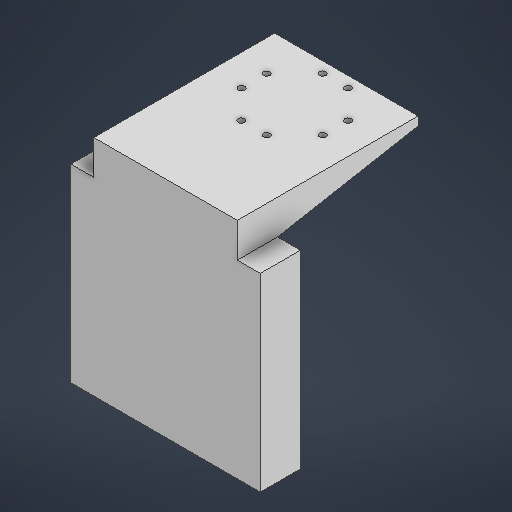
# Autodesk Inventor part: pan_base_holder_third
Saved by Autodesk Inventor 2026 (Build 300175000, 175)
## iProperties
Created: 2025-06-27
Part Number: pan_base_holder_third
Material: Generic
Document SubType Name: Modeling
Designer: user
Density: 1 g/cm^3
Appearance: Default
Author: user
Autodesk Inventor part; units mm, degrees
ref_plane "YZ Plane" through (0, 0, 0) normal (1, 0, 0) x (0, 1, 0)
ref_plane "XZ Plane" through (0, 0, 0) normal (0, 1, 0) x (-1, 0, 0)
ref_plane "XY Plane" through (0, 0, 0) normal (0, 0, 1) x (1, 0, 0)
sketch "Sketch1" plane through (0, 0, 0) normal (0, 0, 1) x (1, 0, 0)
  line L0 (-31, -31) -> (31, -31)
  line L1 (31, -31) -> (31, 31)
  line L2 (31, 31) -> (-31, 31)
  line L3 (-31, 31) -> (-31, -31)
  line L4 (-31, -31) -> (31, 31) construction
  line L5 (31, -31) -> (-31, 31) construction
  line L6 (-33, 33) -> (33, 33)
  line L7 (33, 33) -> (33, -33)
  line L8 (33, -33) -> (-33, -33)
  line L9 (-33, -33) -> (-33, 33)
  point P0 (0, 0)
  dimension "d0" = 62
  dimension "d1" = 62
  dimension "d2" = 2
  constraints: 20 end point, 4 parallel, 2 midpoint, 2 perpendicular, 1 horizontal, 3 other
  measures "d0" distance of L1.end L2.end
  measures "d1" distance of L0.end L1.end
  measures "d2" distance between parallel lines of L2 L6
extrude "Extrusion1" add sketch "Sketch1" along normal blind 2 contours L3 L2 L1 L0 | L6 L7 L8 L9
extrude "Extrusion2" add sketch "Sketch1" against normal blind 12
sketch "Sketch2" plane through (-33, 33, 2) normal (0, 1, 0) x (1, 0, 0)
  line L0 (8, 3) -> (58, 3)
  line L1 (58, 3) -> (58, 0)
  line L2 (58, 0) -> (8, 0)
  line L3 (8, 0) -> (8, 3)
  line L4 (0, 14) -> (0, 0) projected
  line L5 (0, 14) -> (66, 14) projected
  point P0 (33, 2)
  dimension "d7" = 50
  dimension "d8" = 3
  dimension "d9" = 8
  dimension "d10" = 11
  constraints: 8 end point, 2 parallel, 1 horizontal, 1 perpendicular
  measures "d7" distance of L1.end L2.end
  measures "d8" distance of L0.end L1.end
  measures "d9" distance between parallel lines of L4 L3
  measures "d10" distance between parallel lines of L5 L0
extrude "Extrusion3" add sketch "Sketch2" along normal blind 12
sketch "Sketch3" plane through (25, 33, -1) normal (0, 0, -1) x (-1, 0, 0)
  line L0 (50, 12) -> (0, 12) projected
  line L1 (50, 0) -> (50, 12) projected
  line L2 (0, 12) -> (50, 12)
  line L3 (50, 12) -> (50, 9)
  line L4 (50, 9) -> (0, 9)
  line L5 (0, 9) -> (0, 12)
  point P0 (25, -33)
  dimension "d13" = 3
  constraints: 8 end point, 2 parallel, 1 horizontal, 1 perpendicular, 1 point on line
  measures "d13" distance of L2.end L3.end
extrude "Extrusion4" add sketch "Sketch3" along normal blind 60
sketch "Sketch8" plane through (-25, 33, -1) normal (-1, 0, 0) x (0, 0, 1)
  line L0 (0, 9) -> (-60, 9) projected
  line L1 (0, 9) -> (-60, 9)
  line L2 (-60, 9) -> (-60, 0)
  line L3 (-60, 0) -> (0, 0)
  line L4 (0, 0) -> (0, 9)
  line L5 (-60, 9) -> (-10.9892, 0)
  point P0 (1, -33)
  dimension "d43" = 9
  constraints: 10 end point, 2 parallel, 1 horizontal, 1 perpendicular, 1 point on line
  measures "d43" distance of L2.end L1.end
extrude "Extrusion9" add sketch "Sketch8" against normal blind 2 contours L4 L3 L5 L0
ref_plane "Work Plane1" through (0, 33, 2) normal (1, 0, 0) x (0, 0, -1)
mirror "Mirror1" about plane through (0, 33, 2) normal (1, 0, 0) of "Extrusion9"
sketch "Sketch9" plane through (-33, 45, 2) normal (0, 1, 0) x (1, 0, 0)
  circle A0 centre (33, 45) radius 5.5
  circle A1 centre (33, 45) radius 6.45
  circle A2 centre (14.625, 45) radius 2.125
  circle A3 centre (51.375, 45) radius 2.125
  line L0 (14.279, 47.0966) -> (28.2925, 49.4093)
  line L1 (14.2406, 42.9101) -> (28.6201, 40.2652)
  line L2 (51.7217, 47.0965) -> (37.702, 49.4152)
  line L3 (51.7594, 42.9101) -> (37.3799, 40.2652)
  line L4 (33, 45) -> (51.375, 45)
  line L5 (33, 45) -> (14.625, 45)
  circle A4 centre (18.825, 40.6) radius 1.15
  circle A5 centre (47.175, 49.4) radius 1.15
  circle A6 centre (47.175, 45.2183) radius 1.15
  circle A7 centre (18.825, 49.4) radius 1.15
  circle A8 centre (28.6, 30.825) radius 1.15
  circle A9 centre (37.4, 30.825) radius 1.15
  circle A10 centre (32.7817, 59.175) radius 1.15
  circle A11 centre (28.6, 59.175) radius 1.15
  circle A12 centre (47.175, 40.6) radius 1.15
  circle A13 centre (47.175, 49.4) radius 1.15
  circle A14 centre (18.825, 44.7817) radius 1.15
  circle A15 centre (18.825, 40.6) radius 1.15
  circle A16 centre (37.4, 59.175) radius 1.15
  circle A17 centre (28.6, 59.175) radius 1.15
  circle A18 centre (33.2183, 30.825) radius 1.15
  circle A19 centre (37.4, 30.825) radius 1.15
  line L6 (8, 0) -> (58, 0) projected
  line L7 (8, 0) -> (8, 63) projected
  point P0 (33, 2)
  point P1 (7.2363, 31.7405)
  point P2 (37.6183, 45)
  dimension "d48" = 12.9
  dimension "d49" = 4.25
  dimension "d50" = 4.25
  dimension "d51" = 9.15
  dimension "d52" = 9.15
  dimension "d53" = 41
  dimension "d54" = 18.375
  dimension "d55" = 2.3
  dimension "d56" = 4.4
  dimension "d57" = 4.2
  dimension "d58" = 2.3
  dimension "d59" = 4.4
  dimension "d60" = 4.2
  dimension "d62" = 360
  dimension "d64" = 45
  dimension "d67" = 25
  constraints: 20 centre point, 12 end point, 8 point on circle, 4 tangent, 2 coincident, 2 horizontal, 1 collinear, 1 symmetric about line, 34 other
  measures "d48" diameter of A1
  measures "d49" diameter of A2
  measures "d50" diameter of A3
  measures "d51" distance of L1.end L0.end
  measures "d52" vertical distance of L3.end L2.end
  measures "d54" distance of L5.start L5.end
  measures "d55" diameter of A4
  measures "d56" distance from line of L5 A4.centre
  measures "d57" horizontal distance of L5.end A4.centre
  measures "d58" diameter of A5
  measures "d59" distance from line of L4 A5.centre
  measures "d60" horizontal distance of A5.centre L4.end
  measures "d64" distance from line of L6 point (37.618, 45)
  measures "d67" distance from line of L7 point (33, 45)
extrude "Extrusion10" cut sketch "Sketch9" against normal blind 10 contours A4 | A5 | A7 | A8 | A9 | A11 | A12 | A16
body "Solid1"
